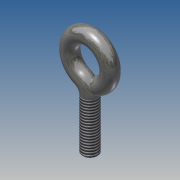
# Autodesk Inventor part: Ösenschraube_M3x15
Saved by Autodesk Inventor 2015 SP1 (Build 190203100, 203)
## iProperties
Created: 2015-03-05
Part Number: Ösenschraube_M3x15
Material: Stahl, galvanisiert
Document SubType Name: Modeling
Designer: Marc
Mass: 1.93933 g
Surface Area: 3.43535 cm^2
Volume: 0.247048 cm^3
Density: 7.85 g/cm^3
Appearance: Galvanisiert
Author: Marc
Autodesk Inventor part; units mm, degrees
ref_plane "YZ Plane" through (0, 0, 0) normal (1, 0, 0) x (0, 1, 0)
ref_plane "XZ Plane" through (0, 0, 0) normal (0, 1, 0) x (-1, 0, 0)
ref_plane "XY Plane" through (0, 0, 0) normal (0, 0, 1) x (1, 0, 0)
sketch "Skizze1" plane through (0, 0, 0) normal (0, 0, 1) x (1, 0, 0)
  line L0 (0, -2.1) -> (0, 2.1) projected
  line L1 (-2.1, 0) -> (2.1, 0) projected
  circle A0 centre (0, 0) radius 1.5
  dimension "d0" = 3
  constraints: 1 centre point, 1 coincident
  measures "d0" diameter of A0
extrude "Extrusion1" add sketch "Skizze1" along normal blind 10
thread "Gewinde1"
sketch "Skizze2" plane through (0, 0, 0) normal (0, 1, 0) x (-1, 0, 0)
  line L0 (0, -2) -> (0, 12) projected
  arc A0 (1.5385, 12.3077) -> (-1.5054, 12.2941) centre (0, 16) ccw
  line L1 (1.5, 10) -> (-1.5, 10) projected
  arc A1 (1.5385, 12.3077) -> (0, 10) centre (2.5, 10) ccw
  point P0 (0, 0)
  dimension "d5" = 8
  dimension "d6" = 6
  constraints: 4 point on circle, 2 centre point, 2 tangent, 1 midpoint, 1 point on line
  measures "d5" diameter of A0
  measures "d6" distance from line of L1 A0.centre
sketch "Skizze3" plane through (0, 0, 10) normal (0, 0, 1) x (1, 0, 0)
  circle A0 centre (0, 0) radius 1.5 projected
sweep "Sweeping1" add profiles "Skizze3" path "Skizze2" path curves A1 A0
chamfer "Fase1" distance 0.2 angle 45 1 edges at (-1.5, 0, 0)
